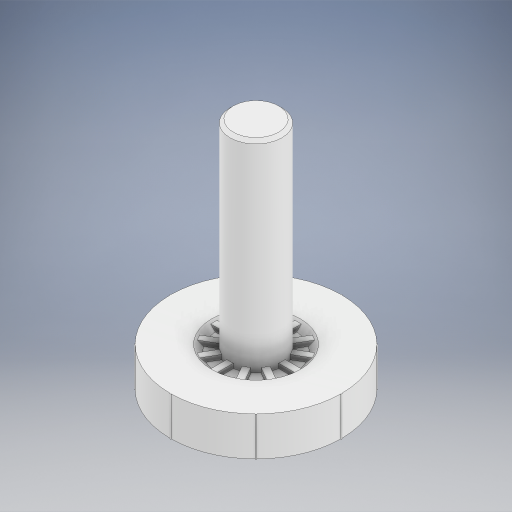
# Autodesk Inventor part: Piston
Saved by Autodesk Inventor 2024.1 (Build 281209000, 209)
## iProperties
Created: 2023-11-09
Part Number: Piston
Material: Acetal Resin, White
Document SubType Name: Modeling
Designer: Glen Collingwood
Density: 1.425 g/cm^3
Appearance: Smooth - White
Author: Glen Collingwood
Autodesk Inventor part; units mm, degrees
ref_plane "YZ Plane" through (0, 0, 0) normal (1, 0, 0) x (0, 1, 0)
ref_plane "XZ Plane" through (0, 0, 0) normal (0, 1, 0) x (-1, 0, 0)
ref_plane "XY Plane" through (0, 0, 0) normal (0, 0, 1) x (1, 0, 0)
sketch "Sketch1" plane through (0, 0, 0) normal (0, 1, 0) x (-1, 0, 0)
  circle A0 centre (0, 0) radius 13.15
  dimension "d0" = 26.3
  constraints: 1 centre point, 1 coincident
  measures "d0" diameter of A0
extrude "Extrusion1" add sketch "Sketch1" along normal blind 6.5
sketch "Sketch2" plane through (0, 0, 0) normal (0, -1, 0) x (1, 0, 0)
  circle A0 centre (0, 0) radius 13.15 projected
  circle A1 centre (0, 0) radius 11.75
  dimension "d3" = 23.5
  constraints: 1 centre point, 1 coincident
  measures "d3" diameter of A1
extrude "Extrusion2" cut sketch "Sketch2" against normal blind 0.5
sketch "Sketch3" plane through (0, 0, 0) normal (0, -1, 0) x (1, 0, 0)
  circle A0 centre (0, 0) radius 11.25
  dimension "d6" = 22.5
  constraints: 1 centre point, 1 coincident
  measures "d6" diameter of A0
extrude "Extrusion3" cut sketch "Sketch3" against normal blind 6
sketch "Sketch4" plane through (0, 6.5, 0) normal (0, 1, 0) x (1, 0, 0)
  circle A0 centre (0, 0) radius 4
  dimension "d9" = 8
  constraints: 1 centre point, 1 coincident
  measures "d9" diameter of A0
extrude "Extrusion4" add sketch "Sketch4" along normal blind 30
chamfer "Chamfer1" distance 0.5 angle 45 1 edges at (-4, 36.5, 0)
sketch "Sketch5" plane through (0, 6, 0) normal (0, -1, 0) x (1, 0, 0)
  circle A0 centre (0, 0) radius 7
  dimension "d15" = 14
  constraints: 1 centre point, 1 coincident
  measures "d15" diameter of A0
extrude "Extrusion5" add sketch "Sketch5" along normal blind 1
chamfer "Chamfer2" distance 1 angle 45 1 edges at (-7, 5, 0)
sketch "Sketch6" plane through (0, 5, 0) normal (0, -1, 0) x (1, 0, 0)
  point P0 (0, 0)
hole "Hole1" at (0, 5, 0) direction (0, 1, 0) diameter 6 depth 30
sketch "Sketch7" plane through (0, 0, 0) normal (1, 0, 0) x (0, 1, 0)
  line L0 (6.5, 4) -> (6.5, -4) projected
  line L1 (6.5, -4) -> (5.5, -4)
  line L2 (5.5, -4) -> (5.5, -5.7929)
  line L3 (5.5, -5.7929) -> (6.5, -6.7929)
  line L4 (6.5, -13.15) -> (6.5, 13.15) projected
  line L5 (0.5, -11.75) -> (0, -11.75) projected
  line L6 (0, -11.75) -> (0, -11.25) projected
  line L7 (0, -11.25) -> (6, -11.25) projected
  line L8 (6, -11.25) -> (6, -7) projected
  line L9 (6, -7) -> (5, -6) projected
  line L10 (5, -6) -> (5, -3) projected
  line L11 (5, -3) -> (35, -3) projected
  line L12 (35, -3) -> (35, 3) projected
  line L13 (35, 3) -> (5, 3) projected
  line L14 (5, 3) -> (5, 6) projected
  line L15 (5, 6) -> (6, 7) projected
  line L16 (6, 7) -> (6, 11.25) projected
  line L17 (6, 11.25) -> (0, 11.25) projected
  line L18 (0, 11.25) -> (0, 11.75) projected
  line L19 (0, 11.75) -> (0.5, 11.75) projected
  line L20 (0.5, 11.75) -> (0.5, 13.15) projected
  line L21 (0.5, 13.15) -> (6.5, 13.15) projected
  line L22 (6.5, 13.15) -> (6.5, 4) projected
  line L23 (6.5, 4) -> (36, 4) projected
  line L24 (36, 4) -> (36.5, 3.5) projected
  line L25 (36.5, 3.5) -> (36.5, -3.5) projected
  line L26 (36.5, -3.5) -> (36, -4) projected
  line L27 (36, -4) -> (6.5, -4) projected
  line L28 (6.5, -4) -> (6.5, -13.15) projected
  line L29 (6.5, -13.15) -> (0.5, -13.15) projected
  line L30 (0.5, -13.15) -> (0.5, -11.75) projected
  line L31 (0, 0) -> (40, 0)
  dimension "d28" = 0.5
  dimension "d29" = 0.5
  dimension "d30" = 0.5
  constraints: 8 end point, 2 horizontal, 1 parallel, 1 perpendicular, 1 point on line
  measures "d28" distance between parallel lines of L4 L8
  measures "d29" distance between parallel lines of L9 L3
  measures "d30" distance between parallel lines of L10 L2
revolve "Revolution1" cut sketch "Sketch7" angle 360 about axis through (0, 0, 0) along (0, 1, 0) contours L4 L3 L2 L1
sketch "Sketch8" plane through (0, 0, 0) normal (1, 0, 0) x (0, 1, 0)
  line L0 (0.5, -11.75) -> (0, -11.75) projected
  line L1 (0, -11.75) -> (0, -11.25) projected
  line L2 (0, -11.25) -> (6, -11.25) projected
  line L3 (6, -11.25) -> (6, -7) projected
  line L4 (6, -7) -> (5, -6) projected
  line L5 (5, -6) -> (5, -3) projected
  line L6 (5, -3) -> (35, -3) projected
  line L7 (35, -3) -> (35, 3) projected
  line L8 (35, 3) -> (5, 3) projected
  line L9 (5, 3) -> (5, 6) projected
  line L10 (5, 6) -> (6, 7) projected
  line L11 (6, 7) -> (6, 11.25) projected
  line L12 (6, 11.25) -> (0, 11.25) projected
  line L13 (0, 11.25) -> (0, 11.75) projected
  line L14 (0, 11.75) -> (0.5, 11.75) projected
  line L15 (0.5, 11.75) -> (0.5, 13.15) projected
  line L16 (0.5, 13.15) -> (6.5, 13.15) projected
  line L17 (6.5, 13.15) -> (6.5, 6.7929) projected
  line L18 (6.5, 6.7929) -> (5.5, 5.7929) projected
  line L19 (5.5, 5.7929) -> (5.5, 4) projected
  line L20 (5.5, 4) -> (36, 4) projected
  line L21 (36, 4) -> (36.5, 3.5) projected
  line L22 (36.5, 3.5) -> (36.5, -3.5) projected
  line L23 (36.5, -3.5) -> (36, -4) projected
  line L24 (36, -4) -> (5.5, -4) projected
  line L25 (5.5, -4) -> (5.5, -5.7929) projected
  line L26 (5.5, -5.7929) -> (6.5, -6.7929) projected
  line L27 (6.5, -6.7929) -> (6.5, -13.15) projected
  line L28 (6.5, -13.15) -> (0.5, -13.15) projected
  line L29 (0.5, -13.15) -> (0.5, -11.75) projected
  line L30 (5.5, -3.5) -> (6.2, -3.5)
  line L31 (6.2, -3.5) -> (6.2, -6.4929)
  line L32 (6.2, -6.4929) -> (5.5, -6.4929)
  line L33 (5.5, -6.4929) -> (5.5, -3.5)
  line L34 (6.5, 6.7929) -> (6.5, -6.7929) projected
  point P0 (0, 0)
  point P1 (5.5, -4)
  dimension "d32" = 0.3
  constraints: 8 end point, 2 parallel, 2 point on line, 1 horizontal, 1 perpendicular
  measures "d32" distance between parallel lines of L34 L31
extrude "Extrusion6" add sketch "Sketch8" along normal mid plane 1 contours L26 L25 L24 L31 | L24 L33 L30 L31
pattern_circular "Circular Pattern1" count 12 over 360 about axis through (0, 6.5, 0) along (0, 1, 0) of "Extrusion6"
sketch "Sketch9" plane through (0, 6.5, 0) normal (0, 1, 0) x (1, 0, 0)
  line L0 (0, 0) -> (0, 13.8998)
  circle A0 centre (0, 0) radius 13.25
  circle A1 centre (0, 0) radius 6.7929 projected
  circle A2 centre (0, 0) radius 4 projected
  circle A3 centre (0, 0) radius 3 projected
  circle A4 centre (0, 0) radius 13.15 projected
  circle A5 centre (0, 13.15) radius 0.1
  dimension "d38" = 26.5
  constraints: 2 centre point, 2 end point, 1 coincident, 1 point on line, 1 tangent, 1 vertical, 1 vertical alignment, 1 other
  measures "d38" diameter of A0
extrude "Extrusion7" add sketch "Sketch9" against normal up to surface (6 mm away) contours A5 A4 L0 | L0 A4 A5 | A4 A5 L0 | L0 A5 A4
pattern_circular "Circular Pattern2" count 8 over 360 about axis through (0, 6.5, 0) along (0, 1, 0) of "Extrusion7"
equation "\"d29\" = d28"
equation "\"d30\" = d28"
body "Solid1"
